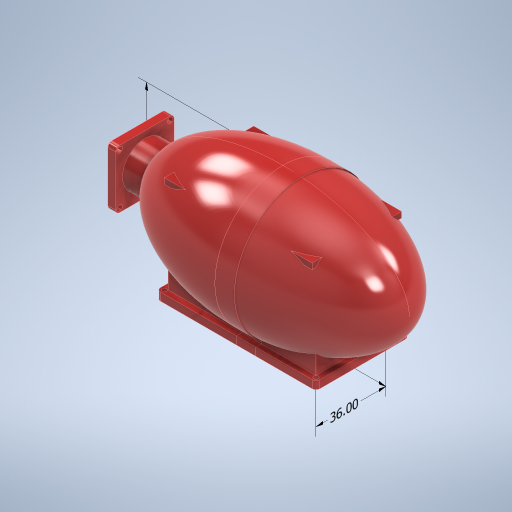
# Autodesk Inventor part: Submarino
Saved by Autodesk Inventor 2023 (Build 270158000, 158)
## iProperties
Created: 2023-03-17
Part Number: Submarino
Material: Plástico PET
Document SubType Name: Modeling
Designer: sergi
Density: 1.541 g/cm^3
Appearance: Rojo naranja
Author: sergi
Autodesk Inventor part; units mm, degrees
note: some values were not read from the file. Chosen so that the rebuilt part matches the saved one: direction of "Agujero2"; direction of "Agujero3"; direction of "Agujero4"; direction of "Agujero5"; direction of "Agujero6"; direction of "Agujero7"; direction of "Agujero8".
ref_plane "XZ Plane" through (0, 0, 0) normal (0, 1, 0) x (-1, 0, 0)
ref_plane "XY Plane" through (0, 0, 0) normal (0, 0, 1) x (1, 0, 0)
sketch "Boceto1" plane through (0, 0, 0) normal (0, 0, 1) x (1, 0, 0)
  line L0 (0, 0) -> (-65, 0)
  line L1 (0, 0) -> (0, 35)
  ellipse E0 centre (0, 0) end of major axis (-65, 0) minor radius 35
  line L2 (0, 0) -> (-62, 0)
  line L3 (0, 0) -> (0, 32)
  ellipse E1 centre (0, 0) end of major axis (-62, 0) minor radius 32
  line L4 (0, 0) -> (65, 0)
  point P0 (62, 0)
  dimension "d0" = 65
  dimension "d1" = 35
  dimension "d2" = 62
  dimension "d3" = 32
  constraints: 10 end point, 4 horizontal, 2 coincident, 2 point on line, 1 vertical, 9 other
  measures "d0" distance of L0.start L0.end
  measures "d1" distance of L0.start L1.end
  measures "d2" distance of L2.start L2.end
  measures "d3" distance of L2.start L3.end
revolve "Revolución1" add sketch "Boceto1" angle 360 about axis through (0, 0, 0) along (-1, 0, 0) contours L0 E0 L1 E1 | L1 E0 L4 E1
sketch "Boceto4" plane through (0, 0, 0) normal (0, 1, 0) x (-1, 0, 0)
  line L0 (-35, -18) -> (35, -18)
  line L1 (35, -18) -> (35, 18)
  line L2 (35, 18) -> (-35, 18)
  line L3 (-35, 18) -> (-35, -18)
  line L4 (-35, -18) -> (35, 18) construction
  line L5 (35, -18) -> (-35, 18) construction
  line L6 (-19.5, -14.5) -> (19.5, 14.5) construction
  line L7 (19.5, -14.5) -> (-19.5, 14.5) construction
  line L8 (-38, -21) -> (38, -21)
  line L9 (38, -21) -> (38, 21)
  line L10 (38, 21) -> (-38, 21)
  line L11 (-38, 21) -> (-38, -21)
  line L12 (-38, -21) -> (38, 21) construction
  line L13 (38, -21) -> (-38, 21) construction
  point P0 (0, 0)
  dimension "d21" = 76
  dimension "d22" = 42
  dimension "d44" = 3
  dimension "d45" = 3
  constraints: 28 end point, 6 midpoint, 4 parallel, 2 horizontal, 2 perpendicular
  measures "d21" distance of L10.end L9.end
  measures "d22" distance of L10.end L8.start
  measures "d44" distance between parallel lines of L10 L2
  measures "d45" distance between parallel lines of L9 L1
extrude "Extrusión1" add sketch "Boceto4" along normal blind 22 and the other way blind 33
extrude "Extrusión2" cut sketch "Boceto4" along normal blind 15 and the other way blind 35 contours L3 L2 L1 L0
sketch "Boceto6" plane through (0, 0, 0) normal (0, 0, 1) x (1, 0, 0)
  point P0 (0, 0)
ref_plane "Plano de trabajo1" through (-60, 0, 0) normal (1, 0, 0) x (0, 1, 0)
sketch "Boceto9" plane through (-60, 0, 0) normal (1, 0, 0) x (0, 1, 0)
  circle A0 centre (0, 0) radius 11.5
  circle A1 centre (0, 0) radius 8.5
  dimension "d46" = 23
  dimension "d49" = 3
  constraints: 2 centre point, 2 coincident
  measures "d46" diameter of A0
  measures "d49" radial gap between concentric circles of A0 A1
extrude "Extrusión5" cut sketch "Boceto9" against normal blind 30 contours A0 | A1
extrude "Extrusión7" cut sketch "Boceto9" along normal blind 10 contours A1
extrude "Extrusión8" add sketch "Boceto9" along normal mid plane 30
sketch "Boceto10" plane through (-75, 0, 0) normal (-1, 0, 0) x (0, 0, 1)
  line L0 (13, -15) -> (-13, -15)
  line L1 (-15, -13) -> (-15, 13)
  line L2 (-13, 15) -> (13, 15)
  line L3 (15, 13) -> (15, -13)
  line L4 (0, 32) -> (0, 0) projected
  line L5 (15, -15) -> (-15, 15) construction
  line L6 (-15, -15) -> (15, 15) construction
  circle A0 centre (0, 0) radius 11.5
  arc A1 (-13, 15) -> (-15, 13) centre (-13, 13) ccw
  arc A2 (-15, -13) -> (-13, -15) centre (-13, -13) ccw
  arc A3 (13, -15) -> (15, -13) centre (13, -13) ccw
  arc A4 (15, 13) -> (13, 15) centre (13, 13) ccw
  point P0 (0, 11.5)
  dimension "d56" = 30
  dimension "d57" = 30
  dimension "d104" = 2
  constraints: 12 end point, 8 point on circle, 8 point on line, 8 tangent, 5 centre point, 3 equal radius, 2 midpoint, 2 parallel, 1 coincident, 1 horizontal, 1 perpendicular
  measures "d56" distance of L5.end L6.end
  measures "d57" distance of L6.start L5.end
  measures "d104" radius of A1
extrude "Extrusión9" add sketch "Boceto10" against normal blind 4
sketch "Boceto12" plane through (0, 22, 0) normal (0, 1, 0) x (1, 0, 0)
  line L0 (-38, 21) -> (38, -21) construction
  line L1 (35, 20) -> (-35, -20) construction
  line L2 (-38, -23) -> (38, -23)
  line L3 (38, -23) -> (38, 23)
  line L4 (38, 23) -> (-38, 23)
  line L5 (-38, 23) -> (-38, -23)
  line L6 (-38, -23) -> (38, 23) construction
  line L7 (38, -23) -> (-38, 23) construction
  point P0 (0, 0)
  dimension "d80" = 76
  dimension "d81" = 46
  constraints: 16 end point, 4 midpoint, 2 parallel, 1 horizontal, 1 perpendicular
  measures "d80" distance of L3.end L4.end
  measures "d81" distance of L4.end L2.start
extrude "Extrusión10" add sketch "Boceto12" against normal blind 3
sketch "Boceto14" plane through (0, -33, 0) normal (0, -1, 0) x (1, 0, 0)
  line L0 (38, 21) -> (-38, 21) projected
  line L1 (38, -21) -> (-38, -21)
  line L2 (-38, -21) -> (-38, 21)
  line L3 (-38, 21) -> (38, 21)
  line L4 (38, 21) -> (38, -21)
  line L5 (38, -21) -> (-38, 21) construction
  line L6 (-38, -21) -> (38, 21) construction
  line L7 (39, -24) -> (-39, -24)
  line L8 (-41, -22) -> (-41, 22)
  line L9 (-39, 24) -> (39, 24)
  line L10 (41, 22) -> (41, -22)
  line L11 (41, -24) -> (-41, 24) construction
  line L12 (-41, -24) -> (41, 24) construction
  arc A0 (-39, 24) -> (-41, 22) centre (-39, 22) ccw
  arc A1 (41, 22) -> (39, 24) centre (39, 22) ccw
  arc A2 (39, -24) -> (41, -22) centre (39, -22) ccw
  arc A3 (-41, -22) -> (-39, -24) centre (-39, -22) ccw
  point P0 (0, 0)
  dimension "d82" = 3
  dimension "d83" = 3
  dimension "d99" = 2
  dimension "d140" = 82
  dimension "d141" = 48
  constraints: 24 end point, 8 point on circle, 8 point on line, 8 tangent, 4 centre point, 4 midpoint, 4 parallel, 3 equal radius, 2 horizontal, 2 perpendicular
  measures "d82" distance between parallel lines of L7 L1
  measures "d83" distance between parallel lines of L10 L4
  measures "d99" radius of A0
  measures "d140" distance between parallel lines of L8 L10
  measures "d141" distance between parallel lines of L9 L7
extrude "Extrusión11" add sketch "Boceto14" against normal blind 4
sketch "Boceto13" plane through (0, 0, 0) normal (0, 0, 1) x (1, 0, 0)
  point P0 (0, 0)
sketch "Boceto16" plane through (0, -33, 0) normal (0, -1, 0) x (1, 0, 0)
  line L0 (-35, 18) -> (35, 18) projected
  line L1 (35, -18) -> (-35, -18)
  line L2 (-35, -18) -> (-35, 18)
  line L3 (-35, 18) -> (35, 18)
  line L4 (35, 18) -> (35, -18)
  line L5 (35, -18) -> (-35, 18) construction
  line L6 (-35, -18) -> (35, 18) construction
  line L7 (-38, -21) -> (38, -21)
  line L8 (38, -21) -> (38, 21)
  line L9 (38, 21) -> (-38, 21)
  line L10 (-38, 21) -> (-38, -21)
  line L11 (-38, -21) -> (38, 21) construction
  line L12 (38, -21) -> (-38, 21) construction
  point P0 (0, 0)
  dimension "d100" = 3
  dimension "d101" = 3
  constraints: 24 end point, 4 midpoint, 4 parallel, 2 horizontal, 2 perpendicular
  measures "d100" distance between parallel lines of L8 L4
  measures "d101" distance between parallel lines of L9 L0
extrude "Extrusión13" cut sketch "Boceto16" against normal blind 1
sketch "Boceto17" plane through (-75, 0, 0) normal (-1, 0, 0) x (0, 0, 1)
  line L0 (10, -10) -> (-10, -10)
  line L1 (-10, -10) -> (-10, 10)
  line L2 (-10, 10) -> (10, 10)
  line L3 (10, 10) -> (10, -10)
  line L4 (0, 32) -> (0, 0) projected
  line L5 (10, -10) -> (-10, 10) construction
  line L6 (-10, -10) -> (10, 10) construction
  line L7 (11, -11) -> (-11, -11)
  line L8 (-11, -11) -> (-11, 11)
  line L9 (-11, 11) -> (11, 11)
  line L10 (11, 11) -> (11, -11)
  line L11 (11, -11) -> (-11, 11) construction
  line L12 (-11, -11) -> (11, 11) construction
  point P0 (0, 11.5)
  dimension "d105" = 1
  dimension "d106" = 1
  dimension "d107" = 10
  constraints: 24 end point, 4 midpoint, 4 parallel, 2 horizontal, 2 perpendicular, 1 point on line
  measures "d105" distance between parallel lines of L9 L2
  measures "d106" distance between parallel lines of L10 L3
  measures "d107" distance from line of L4.end L3
extrude "Extrusión14" cut sketch "Boceto17" against normal blind 1
sketch "Boceto19" plane through (-71, 0, 0) normal (1, 0, 0) x (0, 0, -1)
  point P0 (13, -13)
  point P1 (13, 13)
hole "Agujero2" at (-71, -13, -13) at (-71, 13, -13) direction (-1, 0, 0) diameter 2.9 depth 4
sketch "Boceto20" plane through (-71, 0, 0) normal (1, 0, 0) x (0, 0, -1)
  point P0 (-13, 13)
hole "Agujero3" at (-71, 13, 13) direction (-1, 0, 0) diameter 2.9 depth 4
sketch "Boceto21" plane through (-71, 0, 0) normal (1, 0, 0) x (0, 0, -1)
  point P0 (-13, -13)
hole "Agujero4" at (-71, -13, 13) direction (-1, 0, 0) diameter 2.9 depth 4
sketch "Boceto22" plane through (0, -29, 0) normal (0, 1, 0) x (1, 0, 0)
  point P0 (39, 22)
hole "Agujero5" at (39, -29, -22) direction (0, -1, 0) diameter 2.4 depth 4
sketch "Boceto23" plane through (0, -29, 0) normal (0, 1, 0) x (1, 0, 0)
  point P0 (39, -22)
hole "Agujero6" at (39, -29, 22) direction (0, -1, 0) diameter 2.4 depth 4
sketch "Boceto24" plane through (0, -29, 0) normal (0, 1, 0) x (1, 0, 0)
  point P0 (-39, 22)
hole "Agujero7" at (-39, -29, -22) direction (0, -1, 0) diameter 2.4 depth 4
sketch "Boceto25" plane through (0, -29, 0) normal (0, 1, 0) x (1, 0, 0)
  point P0 (-39, -22)
hole "Agujero8" at (-39, -29, 22) direction (0, -1, 0) diameter 2.4 depth 4
split body "Dividir1" result two bodies by plane through (0, 0, 0) normal (1, 0, 0) first body at (6.8605, 29.4409, -17.6061)
sketch "Boceto26" plane through (0, -32, -18) normal (-1, 0, 0) x (0, 0, 1)
  arc A0 (37, 5.0185) -> (-1, 5.0185) centre (18, 32) ccw
  arc A1 (38, 4.5045) -> (-2, 4.5045) centre (18, 32) ccw
  line L0 (-2, 2) -> (-5.073, 2)
  line L1 (-5.2, -1) -> (-5.2, 3) projected
  line L2 (-5.073, 2) -> (-5.073, -1)
  line L3 (-5.073, -1) -> (-4.073, -1)
  line L4 (-4, -1) -> (40, -1) projected
  line L5 (-4.073, -1) -> (-4.073, 1)
  line L6 (-4.073, 1) -> (-1, 1)
  line L7 (-2, 2) -> (-2, 3)
  line L8 (-1, 1) -> (-1, 2.409)
  line L9 (-6, -1) -> (-3, -1) projected
  line L10 (0, 0) -> (0, 51) projected
  line L11 (-3, 4) -> (-3, 3) projected
  line L12 (-2, 3) -> (-2, 4.5045)
  line L13 (-1, 5.0185) -> (-1, 2.409)
  line L14 (37, 5.0185) -> (37, 1)
  line L15 (37, 1) -> (40, 1)
  line L16 (40, -1) -> (40, 3) projected
  line L17 (40, 1) -> (40, -1)
  line L18 (38, 4.5045) -> (38, 2)
  line L19 (38, 2) -> (41, 2)
  line L20 (41, 2) -> (41, -1)
  line L21 (39, -1) -> (42, -1) projected
  line L22 (40, -1) -> (41, -1)
  line L23 (-3, 3) -> (-6, 3) projected
  line L24 (39, 3) -> (39, 4) projected
  line L25 (42, 3) -> (39, 3) projected
  dimension "d170" = 66
  dimension "d171" = 68
  dimension "d174" = 1
  dimension "d175" = 1
  dimension "d176" = 1
  dimension "d178" = 3
  dimension "d179" = 1
  dimension "d180" = 1
  dimension "d181" = 1
  dimension "d182" = 1
  dimension "d204" = 1
  dimension "d205" = 1
  dimension "d206" = 1
  constraints: 32 end point, 6 perpendicular, 6 vertical, 4 point on circle, 3 collinear, 2 centre point, 2 coincident, 1 point on line
  measures "d170" diameter of A0
  measures "d171" diameter of A1
  measures "d174" distance of L2.end L3.end
  measures "d175" distance between parallel lines of L0 L6
  measures "d176" distance between parallel lines of L7 L8
  measures "d178" distance between parallel lines of L10 L11
  measures "d179" distance between parallel lines of L10 L8
  measures "d180" distance of L4.end L20.end
  measures "d181" distance between parallel lines of L19 L15
  measures "d182" distance between parallel lines of L18 L14
  measures "d204" distance between parallel lines of L23 L0
  measures "d205" distance between parallel lines of L24 L18
  measures "d206" distance between parallel lines of L25 L19
extrude "Extrusión15" add sketch "Boceto26" along normal blind 8 contours A0 L13 L8 L6 L5 L3 L2 L0 L7 L12 A1 L18 L19 L16 L15 L14 | L16 L19 L20 L21 bodies 2
sketch "Boceto27" plane through (0, -32, 18) normal (1, 0, 0) x (0, 0, -1)
  arc A0 (39, 4) -> (-3, 4) centre (18, 32) ccw
  arc A1 (39, 7.8546) -> (-3, 7.8546) centre (18, 32) ccw
  line L0 (-3, 3) -> (-3, 4) projected
  line L1 (-3, 4) -> (-3, 3)
  line L2 (-6, 3) -> (-3, 3) projected
  line L3 (-3, 3) -> (-6, 3)
  line L4 (-6, -1) -> (-6, 3) projected
  line L5 (-6, 3) -> (-6, -1)
  line L6 (40, -1) -> (42, -1) projected
  line L7 (-6, -1) -> (42, -1)
  line L8 (42, -1) -> (42, 3)
  line L9 (39, 12.8865) -> (39, 3) projected
  line L10 (42, 3) -> (39, 3)
  line L11 (39, 3) -> (39, 4)
  line L12 (39, 7.9433) -> (39, 7.8546)
  line L13 (-3, 7.8546) -> (-3, 51.0349)
  line L14 (-3, 51.0349) -> (-3, 54)
  line L15 (0.0466, 54) -> (-5, 54) projected
  line L16 (39, 51.0349) -> (39, 54)
  line L17 (39, 54) -> (0.0466, 54)
  line L18 (-3, 54) -> (0.0466, 54)
  line L19 (39, 51.0349) -> (39, 7.8546)
  line L20 (0, 0) -> (0, 51) projected
  line L21 (36, 0) -> (36, 51) projected
  line L22 (0, 51) -> (36, 51)
  line L23 (36, 51) -> (36, 0)
  line L24 (39, 0) -> (-3, 0) projected
  line L25 (36, 0) -> (39, 0)
  line L26 (39, -1) -> (39, 0) projected
  line L27 (39, 0) -> (39, -1)
  line L28 (39, -1) -> (42, -1)
  line L29 (39, -1) -> (-3, -1) projected
  line L30 (-3, -1) -> (-3, 0)
  line L31 (-3, 0) -> (0, 0)
  line L32 (0, 0) -> (0, 51)
  point P0 (39, 7.8546)
  point P1 (-3, 0)
  dimension "d185" = 70
  dimension "d186" = 64
  constraints: 44 end point, 12 perpendicular, 6 point on line, 4 point on circle, 4 vertical, 2 centre point, 2 coincident, 1 collinear, 1 horizontal, 1 midpoint
  measures "d185" diameter of A0
  measures "d186" diameter of A1
extrude "Extrusión16" add sketch "Boceto27" along normal blind 10 contours L9 L10 L8 L6 L7 L26 L24 L21 L22 L20 L30 L4 L2 L0 A0 bodies 3
sketch "Boceto28" plane through (10, -32, 18) normal (1, 0, 0) x (0, 0, -1)
  arc A0 (37, 5.0185) -> (-1, 5.0185) centre (18, 32) ccw
  arc A1 (38, 4.5045) -> (-2, 4.5045) centre (18, 32) ccw
  line L0 (-2, 4.5045) -> (-2, 2)
  line L1 (-2, 2) -> (-5, 2)
  line L2 (-5, 2) -> (-5, -1)
  line L3 (-6, -1) -> (-3, -1) projected
  line L4 (-5, -1) -> (-4, -1)
  line L5 (-4, -1) -> (-4, 1)
  line L6 (-4, 1) -> (-1, 1)
  line L7 (-1, 1) -> (-1, 5.0185)
  line L8 (-3, 3) -> (-6, 3) projected
  line L9 (-3, 4) -> (-3, 3) projected
  line L10 (37, 5.0185) -> (37, 1)
  line L11 (37, 1) -> (40, 1)
  line L12 (40, 1) -> (40, -1)
  line L13 (40, -1) -> (40, 3) projected
  line L14 (40, -1) -> (41, -1)
  line L15 (41.2, -1) -> (38.8, -1) projected
  line L16 (41, -1) -> (41, 2)
  line L17 (41, 2) -> (38, 2)
  line L18 (38, 2) -> (38, 4.5045)
  line L19 (42, -1) -> (42, 3) projected
  line L20 (42, 3) -> (39, 3) projected
  line L21 (39, 3) -> (39, 4) projected
  point P0 (37, 3.0093)
  dimension "d189" = 66
  dimension "d190" = 68
  dimension "d191" = 1
  dimension "d192" = 1
  dimension "d193" = 1
  dimension "d194" = 1
  dimension "d195" = 1
  dimension "d196" = 1
  dimension "d197" = 1
  dimension "d199" = 1
  dimension "d200" = 1
  dimension "d201" = 1
  dimension "d202" = 1
  dimension "d203" = 1
  constraints: 28 end point, 9 perpendicular, 4 point on circle, 3 point on line, 2 centre point, 2 coincident, 2 vertical, 1 collinear, 1 midpoint
  measures "d189" diameter of A0
  measures "d190" diameter of A1
  measures "d191" distance of L2.end L4.end
  measures "d192" distance of L3.end L4.end
  measures "d193" distance between parallel lines of L1 L6
  measures "d194" distance between parallel lines of L8 L1
  measures "d195" distance between parallel lines of L7 L0
  measures "d196" distance between parallel lines of L9 L0
  measures "d197" distance of L12.end L14.end
  measures "d199" distance between parallel lines of L10 L18
  measures "d200" distance between parallel lines of L17 L11
  measures "d201" distance between parallel lines of L19 L16
  measures "d202" distance between parallel lines of L20 L17
  measures "d203" distance between parallel lines of L21 L18
extrude "Extrusión17" cut sketch "Boceto28" against normal blind 7 bodies 3
